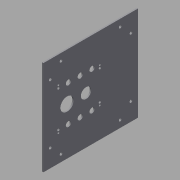
# Autodesk Inventor part: Custom GearBox Mount
Saved by Autodesk Inventor 2013 (Build 170138000, 138)
## iProperties
Created: 2013-01-10
Part Number: Custom GearBox Mount
Material: Generic
Document SubType Name: Modeling
Designer: Naphat
Density: 1 g/cm^3
Author: Naphat
Autodesk Inventor part; units mm, degrees
ref_plane "YZ Plane" through (0, 0, 0) normal (1, 0, 0) x (0, 1, 0)
ref_plane "XZ Plane" through (0, 0, 0) normal (0, 1, 0) x (-1, 0, 0)
ref_plane "XY Plane" through (0, 0, 0) normal (0, 0, 1) x (1, 0, 0)
sketch "Sketch1" plane through (0, 0, 0) normal (1, 0, 0) x (0, 1, 0)
  line L0 (101.6, 101.6) -> (101.6, -101.6)
  line L1 (101.6, -101.6) -> (-101.6, -101.6)
  line L2 (-101.6, -101.6) -> (-101.6, 101.6)
  line L3 (-101.6, 101.6) -> (101.6, 101.6)
  line L4 (-101.6, -101.6) -> (0, -101.6)
  circle A0 centre (63.5, 86.6) radius 3
  circle A1 centre (86.6, 63.5) radius 3
  circle A2 centre (63.5, -86.6) radius 3
  circle A3 centre (86.6, -63.5) radius 3
  circle A4 centre (-63.5, 86.6) radius 3
  circle A5 centre (-86.6, 63.5) radius 3
  circle A6 centre (-63.5, -86.6) radius 3
  circle A7 centre (-86.6, -63.5) radius 3
  circle A8 centre (-50.8, 0) radius 14.2875
  circle A9 centre (-9.965, 0) radius 11.1125
  circle A10 centre (-22.513, -38.7346) radius 5.5563
  circle A11 centre (-22.5126, 38.7346) radius 5.5563
  circle A12 centre (-47.9139, -38.7346) radius 5.5562
  circle A13 centre (2.8879, -38.7346) radius 5.5563
  circle A14 centre (2.8874, 38.7346) radius 5.5563
  circle A15 centre (-47.9126, 38.7346) radius 5.5563
  point P0 (0, 0)
  dimension "d28" = 28.575
  dimension "d30" = 22.225
  dimension "d39" = 6
  dimension "d42" = 38.1
  dimension "d43" = 38.1
  dimension "d44" = 38.1
  dimension "d45" = 38.1
  dimension "d46" = 15
  dimension "d47" = 38.1
  dimension "d49" = 15
  dimension "d50" = 15
  dimension "d51" = 15
  dimension "d52" = 38.1
  dimension "d53" = 15
  dimension "d57" = 101.6
  dimension "d58" = 50.8
  dimension "d60" = 40.835
  dimension "d61" = 203.2
  dimension "d62" = 203.2
  dimension "d63" = 101.6
  dimension "d64" = 101.6
  dimension "d65" = 91.635
  dimension "d66" = 38.1
  dimension "d67" = 38.1
  dimension "d68" = 15
  dimension "d69" = 15
  dimension "d70" = 15
  dimension "d71" = 101.6
  dimension "d72" = 101.6
  dimension "d91" = 11.1125
  dimension "d99" = 53.6861
  dimension "d100" = 25.4009
  dimension "d101" = 25.4009
  constraints: 16 centre point, 10 end point, 7 equal radius, 2 horizontal alignment, 2 parallel, 1 midpoint, 1 perpendicular, 1 vertical
  measures "d28" diameter of A8
  measures "d30" diameter of A9
  measures "d39" diameter of A5
  measures "d42" distance from line of A4.centre L2
  measures "d43" distance from line of L3 A5.centre
  measures "d44" distance from line of L3 A1.centre
  measures "d45" distance from line of A0.centre L0
  measures "d46" distance from line of L0 A3.centre
  measures "d47" distance from line of A3.centre L1
  measures "d49" distance from line of A6.centre L1
  measures "d50" distance from line of A2.centre L1
  measures "d51" distance from line of A7.centre L2
  measures "d52" distance from line of L2 A6.centre
  measures "d53" distance from line of L2 A5.centre
  measures "d57" distance from line of point (0, 0) L0
  measures "d58" distance from line of A8.centre L2
  measures "d60" distance of A9.centre A8.centre
  measures "d61" distance of L0.start L0.end
  measures "d62" distance of L0.end L1.end
  measures "d63" distance from line of L1 A8.centre
  measures "d64" distance from line of L4 A9.centre
  measures "d65" distance from line of L2 A9.centre
  measures "d66" distance from line of L4 A7.centre
  measures "d67" distance from line of A2.centre L0
  measures "d68" distance from line of L0 A1.centre
  measures "d69" distance from line of L3 A0.centre
  measures "d70" distance from line of L3 A4.centre
  measures "d71" distance from line of point (0, 0) L3
  measures "d72" distance from line of L4.end L0
  measures "d91" diameter of A13
  measures "d99" distance from line of L2 A12.centre
  measures "d100" distance of A12.centre A10.centre
  measures "d101" distance of A10.centre A13.centre
ref_plane "Work Plane1" through (0, 0, 0) normal (1, 0, 0) x (0, 0, -1)
extrude "Extrusion4" add sketch "Sketch1" along normal blind 3
sketch "Sketch3" plane through (0, 0, 0) normal (-1, 0, 0) x (0, 0, 1)
  circle A0 centre (0, -50.8) radius 14.2875 projected
  circle A1 centre (0, -9.965) radius 11.1125 projected
  line L0 (101.6, -101.6) -> (-101.6, -101.6) projected
  line L1 (0, -50.8) -> (38.735, -50.8) construction
  line L2 (38.735, -50.8) -> (38.735, -69.112) construction
  circle A2 centre (38.735, -69.112) radius 2.5525
  line L3 (38.735, -69.112) -> (44.577, -69.112) construction
  circle A3 centre (44.577, -69.112) radius 2.0445
  line L4 (44.577, -69.112) -> (-44.577, -69.112) construction
  circle A4 centre (-44.577, -69.112) radius 2.0445
  line L5 (-44.577, -69.112) -> (-38.735, -69.112) construction
  circle A5 centre (-38.735, -69.112) radius 2.5525
  line L6 (0, -9.965) -> (37.592, -9.965) construction
  line L7 (37.592, -9.965) -> (37.592, 19.907) construction
  circle A6 centre (37.592, 19.907) radius 2.0445
  line L8 (37.592, 19.907) -> (31.75, 19.907) construction
  circle A7 centre (31.75, 19.907) radius 2.5525
  line L9 (37.592, 19.907) -> (-37.592, 19.907) construction
  circle A8 centre (-37.592, 19.907) radius 2.0445
  line L10 (-37.592, 19.907) -> (-31.75, 19.907) construction
  circle A9 centre (-31.75, 19.907) radius 2.5525
  point P0 (0, 0)
  dimension "d104" = 38.735
  dimension "d105" = 18.312
  dimension "d106" = 5.105
  dimension "d107" = 5.842
  dimension "d108" = 4.089
  dimension "d109" = 89.154
  dimension "d110" = 4.089
  dimension "d111" = 5.842
  dimension "d112" = 5.105
  dimension "d113" = 37.592
  dimension "d114" = 29.872
  dimension "d115" = 4.089
  dimension "d116" = 5.842
  dimension "d117" = 5.105
  dimension "d118" = 75.184
  dimension "d119" = 5.842
  dimension "d120" = 4.089
  dimension "d121" = 5.105
  constraints: 20 end point, 8 centre point, 8 coincident, 4 perpendicular, 2 collinear, 2 parallel, 2 point on line
  measures "d104" distance of L1.start L1.end
  measures "d105" distance of L1.end L2.end
  measures "d106" diameter of A2
  measures "d107" distance of L3.start L3.end
  measures "d108" diameter of A3
  measures "d109" distance of L4.start L4.end
  measures "d110" diameter of A4
  measures "d111" distance of L5.start L5.end
  measures "d112" diameter of A5
  measures "d113" distance of L6.start L6.end
  measures "d114" distance of L6.end L7.end
  measures "d115" diameter of A6
  measures "d116" distance of L8.start L8.end
  measures "d117" diameter of A7
  measures "d118" distance of L8.start L9.end
  measures "d119" distance of L10.start L10.end
  measures "d120" diameter of A8
  measures "d121" diameter of A9
extrude "Extrusion5" cut sketch "Sketch3" against normal blind 10 contours A2 | A3 | A4 | A5 | A6 | A7 | A8 | A9
equation "\"d43\" = d42"
equation "\"d44\" = d43"
equation "\"d45\" = d42"
equation "\"d47\" = d44"
equation "\"d49\" = d46"
equation "\"d50\" = d46"
equation "\"d51\" = d50"
equation "\"d52\" = d42"
equation "\"d53\" = d51"
equation "\"d57\" = 0.5 * d62"
equation "\"d61\" = d62"
equation "\"d63\" = d57"
equation "\"d64\" = d63"
equation "\"d66\" = d43"
equation "\"d67\" = d47"
equation "\"d68\" = d50"
equation "\"d69\" = d68"
equation "\"d70\" = d53"
body "Solid3"
